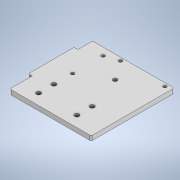
# Autodesk Inventor part: EboxBottom_2
Saved by Autodesk Inventor 2021 (Build 250183000, 183)
## iProperties
Created: 2022-01-03
Part Number: EboxBottom_2
Material: Generic
Document SubType Name: Modeling
Designer: Jorian Brusind
Density: 1 g/cm^3
Appearance: Default
Author: Jorian Brusind
Autodesk Inventor part; units mm, degrees
ref_plane "YZ Plane" through (0, 0, 0) normal (1, 0, 0) x (0, 1, 0)
ref_plane "XZ Plane" through (0, 0, 0) normal (0, 1, 0) x (-1, 0, 0)
ref_plane "XY Plane" through (0, 0, 0) normal (0, 0, 1) x (1, 0, 0)
sketch "Sketch1" plane through (0, 0, 0) normal (0, 1, 0) x (-1, 0, 0)
  line L0 (232.1908, -176.5808) -> (232.1908, -3.7592)
  arc A0 (232.1908, -3.7592) -> (227.4316, 1) centre (227.4316, -3.7592) ccw
  line L1 (227.4316, 1) -> (0, 1)
  arc A1 (0, 1) -> (-4.7592, -3.7592) centre (0, -3.7592) ccw
  arc A2 (-4.7592, -176.5808) -> (0, -181.34) centre (0, -176.5808) ccw
  arc A3 (227.4316, -181.34) -> (232.1908, -176.5808) centre (227.4316, -176.5808) ccw
  circle A4 centre (130, -129.34) radius 2.25
  circle A5 centre (129.9861, -89.34) radius 2.25
  circle A6 centre (90, -129.34) radius 2.25
  circle A7 centre (89.9861, -89.34) radius 2.25
  circle A8 centre (180, -110) radius 2.75
  circle A9 centre (55, -110) radius 2.75
  circle A10 centre (90, -45) radius 3
  circle A11 centre (190, -45) radius 3
  circle A12 centre (190, -65) radius 3
  circle A13 centre (90, -65) radius 3
  circle A14 centre (140, -45) radius 3
  circle A15 centre (40, -45) radius 3
  circle A16 centre (140, -65) radius 3
  circle A17 centre (40, -65) radius 3
  line L2 (230.1908, -176.5808) -> (230.1908, -3.7592)
  arc A18 (230.1908, -3.7592) -> (227.4316, -1) centre (227.4316, -3.7592) ccw
  line L3 (227.4316, -1) -> (0, -1)
  arc A19 (0, -1) -> (-2.7592, -3.7592) centre (0, -3.7592) ccw
  arc A20 (-2.7592, -176.5808) -> (0, -179.34) centre (0, -176.5808) ccw
  arc A21 (227.4316, -179.34) -> (230.1908, -176.5808) centre (227.4316, -176.5808) ccw
  line L4 (-4.7592, -3.7592) -> (-4.7592, -176.5808)
  line L5 (-2.7592, -3.7592) -> (-2.7592, -176.5808)
  line L6 (0, -179.34) -> (227.4316, -179.34)
  line L7 (227.4316, -181.34) -> (0, -181.34)
  line L8 (0, 0) -> (0, -15)
  line L9 (0, 0) -> (15, 0) construction
  line L10 (0, 0) -> (15, 0)
  line L11 (0, 0) -> (15, 0) construction
  circle A22 centre (15, -135) radius 2.25
  circle A23 centre (73, -135) radius 2.25
  point P0 (230.1908, -3.7592)
  point P1 (0, -1)
  dimension "d0" = 2
  dimension "d1" = 2
  dimension "d2" = 2
  dimension "d3" = 2
  dimension "d5" = 2
  dimension "d7" = 2
  dimension "d8" = 227.4316
  dimension "d9" = 172.8216
  dimension "d10" = 4.7592
  dimension "d45" = 15
  dimension "d46" = 90
  dimension "d47" = 15
  dimension "d48" = 0
  dimension "d49" = 110
  dimension "d50" = 55
  dimension "d51" = 125
  dimension "d52" = 110
  dimension "d54" = 40
  dimension "d55" = 40
  dimension "d56" = 40
  dimension "d57" = 40
  dimension "d58" = 50
  dimension "d59" = 100.1908
  dimension "d60" = 2.7592
  dimension "d61" = 1
  dimension "d62" = 4.7592
  dimension "d63" = 178.34
  dimension "d64" = 180.34
  dimension "d65" = 172.8216
  dimension "d66" = 230.1908
  dimension "d67" = 4.5
  dimension "d68" = 5.5
  dimension "d69" = 6
  dimension "d70" = 40.1908
  dimension "d71" = 64
  dimension "d72" = 20
  dimension "d73" = 50
  dimension "d74" = 50
  dimension "d75" = 50
  dimension "d76" = 20
  dimension "d77" = 20
  dimension "d78" = 20
  dimension "d79" = 50
  dimension "d87" = 4.5
  dimension "d89" = 25
  dimension "d90" = 40
  dimension "d91" = 4.5
  dimension "d92" = 58
  constraints: 24 centre point, 24 end point, 16 point on circle, 11 equal radius, 7 equal length, 6 horizontal alignment, 3 horizontal, 3 vertical alignment, 2 vertical, 1 tangent
  measures "d0" distance between parallel lines of L0 L2
  measures "d1" radial gap between concentric circles of A0 A18
  measures "d2" distance between parallel lines of L1 L3
  measures "d3" radial gap between concentric circles of A1 A19
  measures "d5" radial gap between concentric circles of A2 A20
  measures "d7" radial gap between concentric circles of A3 A21
  measures "d8" distance of L7.start L7.end
  measures "d9" distance of L0.start L0.end
  measures "d10" radius of A3
  measures "d45" distance of L8.start L8.end
  measures "d46" angle of L8 L9
  measures "d47" distance of L8.start L9.end
  measures "d48" distance between parallel lines of L10 L11
  measures "d49" distance from line of A9.centre L9
  measures "d50" distance from line of A9.centre L8
  measures "d51" distance of A9.centre A8.centre
  measures "d52" distance from line of L10 A8.centre
  measures "d54" distance of A6.centre A4.centre
  measures "d55" distance of A5.centre A4.centre
  measures "d56" distance of A7.centre A5.centre
  measures "d57" distance of A6.centre A7.centre
  measures "d58" distance from line of L6 A4.centre
  measures "d59" distance from line of L2 A4.centre
  measures "d60" distance between parallel lines of L8 L5
  measures "d61" distance between parallel lines of L9 L3
  measures "d62" distance from line of L8.end L4
  measures "d63" distance between parallel lines of L3 L6
  measures "d64" distance between parallel lines of L3 L7
  measures "d65" distance of L2.start L2.end
  measures "d66" distance between parallel lines of L8 L2
  measures "d67" diameter of A4
  measures "d68" diameter of A9
  measures "d69" diameter of A12
  measures "d70" distance from line of L2 A12.centre
  measures "d71" distance from line of L3 A12.centre
  measures "d72" distance of A11.centre A12.centre
  measures "d73" distance of A16.centre A12.centre
  measures "d74" distance of A13.centre A16.centre
  measures "d75" distance of A17.centre A13.centre
  measures "d76" distance of A14.centre A16.centre
  measures "d77" distance of A10.centre A13.centre
  measures "d78" distance of A15.centre A17.centre
  measures "d79" distance of A15.centre A10.centre
  measures "d87" diameter of A22
  measures "d89" vertical distance of A9.centre A22.centre
  measures "d90" horizontal distance of A9.centre A22.centre
  measures "d91" diameter of A23
  measures "d92" distance of A22.centre A23.centre
extrude "Extrusion1" add sketch "Sketch1" along normal blind 6 contours A21 L6 A20 L5 A19 L3 A18 L2
sketch "Sketch2" plane through (0, 6, 0) normal (0, 1, 0) x (1, 0, 0)
  line L0 (-232.1908, 176.5808) -> (-232.1908, 3.7592)
  arc A0 (-232.1908, 3.7592) -> (-227.4316, -1) centre (-227.4316, 3.7592) ccw
  line L1 (-227.4316, -1) -> (0, -1)
  arc A1 (0, -1) -> (4.7592, 3.7592) centre (0, 3.7592) ccw
  arc A2 (4.7592, 176.5808) -> (0, 181.34) centre (0, 176.5808) ccw
  arc A3 (-227.4316, 181.34) -> (-232.1908, 176.5808) centre (-227.4316, 176.5808) ccw
  circle A4 centre (-130, 135) radius 2
  circle A5 centre (-130, 95) radius 2
  circle A6 centre (-90, 135) radius 2
  circle A7 centre (-90, 95) radius 2
  circle A8 centre (-160.0797, 100) radius 2.75
  circle A9 centre (-60.0797, 100) radius 2.75
  circle A10 centre (-90, 45) radius 2.5
  circle A11 centre (-190, 45) radius 2.5
  circle A12 centre (-190, 65) radius 2.5
  circle A13 centre (-90, 65) radius 2.5
  circle A14 centre (-140, 45) radius 2.5
  circle A15 centre (-40, 45) radius 2.5
  circle A16 centre (-140, 65) radius 2.5
  circle A17 centre (-40, 65) radius 2.5
  line L2 (-230.1908, 176.5808) -> (-230.1908, 3.7592)
  arc A18 (-230.1908, 3.7592) -> (-227.4316, 1) centre (-227.4316, 3.7592) ccw
  line L3 (-227.4316, 1) -> (0, 1)
  arc A19 (0, 1) -> (2.7592, 3.7592) centre (0, 3.7592) ccw
  arc A20 (2.7592, 176.5808) -> (0, 179.34) centre (0, 176.5808) ccw
  arc A21 (-227.4316, 179.34) -> (-230.1908, 176.5808) centre (-227.4316, 176.5808) ccw
  line L4 (4.7592, 3.7592) -> (4.7592, 176.5808)
  line L5 (2.7592, 3.7592) -> (2.7592, 176.5808)
  line L6 (0, 179.34) -> (-227.4316, 179.34)
  line L7 (-227.4316, 181.34) -> (0, 181.34)
  line L8 (0, 179.34) -> (-227.4316, 179.34) projected
  line L9 (-113.7158, 179.34) -> (-113.7158, 1)
  line L10 (-227.4316, 1) -> (0, 1) projected
  line L11 (-118.7158, 120.17) -> (-108.7158, 120.17)
  line L12 (-108.7158, 120.17) -> (-108.7158, 60.17)
  line L13 (-108.7158, 60.17) -> (-118.7158, 60.17)
  line L14 (-118.7158, 60.17) -> (-118.7158, 120.17)
  line L15 (-118.7158, 120.17) -> (-108.7158, 60.17) construction
  line L16 (-108.7158, 120.17) -> (-118.7158, 60.17) construction
  line L17 (-113.7158, 179.34) -> (-113.7158, 159.34)
  line L18 (2.7592, 139.34) -> (-230.1908, 139.34)
  line L19 (-230.1908, 139.34) -> (-230.1908, 179.34)
  line L20 (-230.1908, 179.34) -> (2.7592, 179.34)
  line L21 (2.7592, 179.34) -> (2.7592, 139.34)
  line L22 (2.7592, 139.34) -> (-230.1908, 179.34) construction
  line L23 (-230.1908, 139.34) -> (2.7592, 179.34) construction
  line L24 (-113.7158, 1) -> (-113.7158, 16)
  line L25 (-230.1908, 31) -> (2.7592, 31)
  line L26 (2.7592, 31) -> (2.7592, 1)
  line L27 (2.7592, 1) -> (-230.1908, 1)
  line L28 (-230.1908, 1) -> (-230.1908, 31)
  line L29 (-230.1908, 31) -> (2.7592, 1) construction
  line L30 (2.7592, 31) -> (-230.1908, 1) construction
  line L31 (-227.4316, 1) -> (0, 1) projected
  line L32 (-230.1908, 179.34) -> (-200.1908, 179.34)
  line L33 (-200.1908, 179.34) -> (-200.1908, 1)
  line L34 (-200.1908, 1) -> (-230.1908, 1)
  line L35 (-230.1908, 1) -> (-230.1908, 179.34)
  line L36 (2.7592, 1) -> (-7.2408, 1)
  line L37 (-7.2408, 1) -> (-7.2408, 179.34)
  line L38 (-7.2408, 179.34) -> (2.7592, 179.34)
  line L39 (2.7592, 179.34) -> (2.7592, 1)
  point P0 (230.1908, -176.5808)
  point P1 (230.1908, -3.7592)
  point P2 (227.4316, -1)
  point P3 (0, -1)
  point P4 (0, 0)
  point P5 (230.1908, -176.5808)
  point P6 (230.1908, -3.7592)
  point P7 (227.4316, -1)
  point P8 (0, -1)
  point P9 (-113.7158, 90.17)
  point P10 (-113.7158, 120.17)
  point P11 (-113.7158, 60.17)
  point P12 (-113.7158, 1)
  point P13 (0, 1)
  point P14 (-230.1908, 3.7592)
  point P15 (-227.4316, 1)
  point P16 (-113.7158, 139.34)
  point P17 (-7.2408, 139.34)
  point P18 (-7.2408, 31)
  point P19 (-113.7158, 31)
  dimension "d22" = 2
  dimension "d23" = 2
  dimension "d24" = 2
  dimension "d25" = 2
  dimension "d26" = 2
  dimension "d27" = 2
  dimension "d28" = 227.4316
  dimension "d29" = 172.8216
  dimension "d30" = 4.7592
  dimension "d31" = 10
  dimension "d32" = 60
  dimension "d37" = 20
  dimension "d38" = 40
  dimension "d39" = 15
  dimension "d40" = 30
  dimension "d41" = 30
  dimension "d42" = 10
  constraints: 74 end point, 22 centre point, 16 point on circle, 14 parallel, 9 midpoint, 5 horizontal, 5 perpendicular, 4 point on line, 1 tangent
  measures "d22" distance between parallel lines of L0 L2
  measures "d23" radial gap between concentric circles of A0 A18
  measures "d24" distance between parallel lines of L1 L3
  measures "d25" radial gap between concentric circles of A1 A19
  measures "d26" radial gap between concentric circles of A2 A20
  measures "d27" radial gap between concentric circles of A3 A21
  measures "d28" distance of L7.start L7.end
  measures "d29" distance of L0.start L0.end
  measures "d30" radius of A3
  measures "d31" distance of L12.end L13.end
  measures "d32" distance of L11.end L12.end
  measures "d37" distance of L9.start L17.end
  measures "d38" distance of L18.end L19.end
  measures "d39" distance of L9.end L24.end
  measures "d40" distance of L25.end L26.end
  measures "d41" distance of L33.end L34.end
  measures "d42" distance of L37.end L38.end
extrude "Extrusion3" cut sketch "Sketch2" against normal through all contours A4 | A5 | A8 | A11 | A12 | A14 | A16 | A21 L6 L33 L18 L2 | L18 L33 L25 L2 | L25 L33 L3 A18 L2 | L33 L6 L9 L18 | L18 L9 L11 L14 L13 L25 L33 | L25 L9 L3 L33 | L9 L6 L37 L18 | L25 L37 L3 L9 | L37 L6 A20 L5 L18 | L18 L5 L25 L37 | L25 L5 A19 L3 L37
fillet "Fillet3" radius 2 6 edges at (-113.7158, 3, -31) (-118.7158, 3, -60.17) (-118.7158, 3, -120.17) (-7.2408, 3, -31) (-7.2408, 3, -139.34) (-113.7158, 3, -139.34)
equation "\"d1\" = d0"
equation "\"d2\" = d0"
equation "\"d3\" = d0"
equation "\"d5\" = d0"
equation "\"d7\" = d0"
equation "\"d23\" = d22"
equation "\"d24\" = d22"
equation "\"d25\" = d22"
equation "\"d26\" = d22"
equation "\"d27\" = d22"
body "Solid1"
